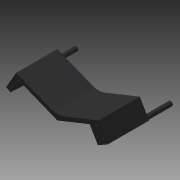
# Autodesk Inventor part: Front Support
Saved by Autodesk Inventor 2015 (Build 190159000, 159)
## iProperties
Created: 2015-11-27
Part Number: Front Support
Material: ABS Plastic
Document SubType Name: Modeling
Designer: James
Density: 1.06 g/cm^3
Appearance: Smooth - White
Mass: 34.4011 g
Surface Area: 179.359 cm^2
Volume: 32.4539 cm^3
Author: James
Autodesk Inventor part; units mm, degrees
ref_plane "YZ Plane" through (0, 0, 0) normal (1, 0, 0) x (0, 1, 0)
ref_plane "XZ Plane" through (0, 0, 0) normal (0, 1, 0) x (-1, 0, 0)
ref_plane "XY Plane" through (0, 0, 0) normal (0, 0, 1) x (1, 0, 0)
sketch "Sketch1" plane through (0, 0, 0) normal (0, 1, 0) x (-1, 0, 0)
  line L0 (56.9199, 1.0144) -> (62.116, 4.0144)
  line L1 (62.116, 4.0144) -> (50, 25)
  line L2 (-50, 25) -> (-61.25, 5.5144)
  line L3 (0.7428, 5.2971) -> (50, 25)
  line L4 (-0.7428, 5.2971) -> (-50, 25)
  line L5 (42.5883, 14.6502) -> (56.9199, 1.0144)
  line L6 (-0.7428, 5.2971) -> (0, 5)
  line L7 (0.7428, 5.2971) -> (0, 5)
  circle A0 centre (47.5441, 18.66) radius 1.4
  circle A1 centre (55.9574, 8.1656) radius 1.4
  circle A2 centre (-55.9574, 8.1656) radius 1.4
  circle A3 centre (-47.5441, 18.66) radius 1.4
  line L8 (-39.2213, 15.6885) -> (0, 0)
  line L9 (42.5883, 14.6502) -> (40.8234, 16.3294)
  line L10 (40.8234, 16.3294) -> (0, 0)
  line L11 (-61.25, 5.5144) -> (-49.134, -1.4808)
  line L12 (-49.134, -1.4808) -> (-39.2213, 15.6885)
  point P0 (0, 0)
  dimension "d0" = 2.8
  dimension "d1" = 2.8
  dimension "d2" = 2.8
  dimension "d3" = 2.8
  dimension "d14" = 5
  constraints: 26 end point, 4 centre point
  measures "d0" diameter of A0
  measures "d1" diameter of A1
  measures "d2" diameter of A2
  measures "d3" diameter of A3
  measures "d14" distance of L6.end L8.end
extrude "Extrusion1" add sketch "Sketch1" along normal blind 50
sketch "Sketch2" plane through (0, 50, 0) normal (0, 1, 0) x (1, 0, 0)
  circle A0 centre (47.5441, -18.66) radius 1.4 projected
  circle A1 centre (55.9574, -8.1656) radius 1.4 projected
  circle A2 centre (-55.9574, -8.1656) radius 1.4 projected
  circle A3 centre (-47.5441, -18.66) radius 1.4 projected
  line L0 (-40.8234, -16.3294) -> (-56.9199, -1.0144) projected
  line L1 (-56.9199, -1.0144) -> (-62.116, -4.0144) projected
  line L2 (-62.116, -4.0144) -> (-50, -25) projected
  line L3 (-50, -25) -> (0, -5) projected
  line L4 (0, -5) -> (50, -25) projected
  line L5 (50, -25) -> (61.25, -5.5144) projected
  line L6 (39.2213, -15.6885) -> (0, 0) projected
  line L7 (0, 0) -> (-40.8234, -16.3294) projected
  line L8 (61.25, -5.5144) -> (49.134, 1.4808) projected
  line L9 (49.134, 1.4808) -> (39.2213, -15.6885) projected
  point P0 (0, 0)
extrude "Extrusion2" add sketch "Sketch2" against normal blind 40 contours A0 | A1 | A2 | A3
sketch "Sketch3" plane through (0, 50, 0) normal (0, 1, 0) x (1, 0, 0)
  line L0 (-62.116, -4.0144) -> (-58.116, -4.0144) construction
  circle A0 centre (-57.3863, -6.5497) radius 1.4
  line L1 (61.25, -5.5144) -> (57.25, -5.5144) construction
  circle A1 centre (57.3863, -6.5497) radius 1.4
  circle A2 centre (57.3863, -6.5497) radius 2.75
  circle A3 centre (-57.3863, -6.5497) radius 2.75
  point P0 (0, 0)
  dimension "d10" = 2.8
  dimension "d15" = 2.8
  dimension "d16" = 5.5
  dimension "d17" = 5.5
  constraints: 4 centre point, 4 end point, 2 coincident, 1 horizontal
  measures "d10" diameter of A0
  measures "d15" diameter of A1
  measures "d16" diameter of A2
  measures "d17" diameter of A3
extrude "Extrusion3" add sketch "Sketch3" along normal blind 30
fillet "Fillet1" radius 20 1 edges at (0, 25, 5)
body "Solid1"
